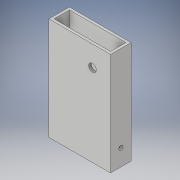
# Autodesk Inventor part: bumper extrusions
Saved by Autodesk Inventor 2019 (Build 230136000, 136)
## iProperties
Created: 2018-12-24
Part Number: bumper extrusions
Material: Generic
Document SubType Name: Modeling
Designer: Tiberus
Density: 1 g/cm^3
Appearance: Default
Author: Tiberus
Autodesk Inventor part; units mm, degrees
ref_plane "YZ Plane" through (0, 0, 0) normal (1, 0, 0) x (0, 1, 0)
ref_plane "XZ Plane" through (0, 0, 0) normal (0, 1, 0) x (-1, 0, 0)
ref_plane "XY Plane" through (0, 0, 0) normal (0, 0, 1) x (1, 0, 0)
sketch "Sketch1" plane through (0, 0, 0) normal (0, 0, 1) x (1, 0, 0)
  line L0 (0, 0) -> (76.2, 0)
  line L1 (76.2, 0) -> (76.2, 127)
  line L2 (76.2, 127) -> (0, 127)
  line L3 (0, 127) -> (0, 0)
  dimension "d0" = 76.2
  dimension "d1" = 127
  constraints: 8 end point, 2 parallel, 1 horizontal, 1 perpendicular
  measures "d0" distance of L2.end L1.end
  measures "d1" distance of L1.end L0.end
extrude "Extrusion1" add sketch "Sketch1" along normal blind 25.4
sketch "Sketch2" plane through (76.2, 0, 0) normal (1, 0, 0) x (0, 0, -1)
  line L0 (0, 0) -> (-25.4, 0) construction
  line L1 (-12.7, 0) -> (-12.7, 20.6502) construction
  circle A0 centre (-12.7, 20.6502) radius 2.5797
  dimension "d4" = 20.6502
  dimension "d5" = 5.1594
  constraints: 2 end point, 1 centre point, 1 coincident, 1 midpoint, 1 vertical
  measures "d4" distance of L1.start L1.end
  measures "d5" diameter of A0
extrude "Extrusion2" cut sketch "Sketch2" against normal blind 762
sketch "Sketch4" plane through (0, 0, 0) normal (0, -1, 0) x (1, 0, 0)
  line L0 (0, 25.4) -> (76.2, 25.4) projected
  line L1 (0, 0) -> (0, 25.4) projected
  line L2 (0, 0) -> (76.2, 0) projected
  line L3 (76.2, 0) -> (76.2, 25.4) projected
  line L4 (73.025, 22.225) -> (3.175, 22.225)
  line L5 (3.175, 22.225) -> (3.175, 3.175)
  line L6 (3.175, 3.175) -> (73.025, 3.175)
  line L7 (73.025, 3.175) -> (73.025, 22.225)
  dimension "d15" = 3.175
  constraints: 8 end point, 3 other
  measures "d15" distance between parallel lines of L0 L4
extrude "Extrusion3" cut sketch "Sketch4" against normal blind 508 contours L7 L6 L5 L4
sketch "Sketch5" plane through (0, 0, 0) normal (-1, 0, 0) x (0, 0, 1)
  line L0 (0, 127) -> (25.4, 127) construction
  line L1 (12.7, 127) -> (12.7, 114.3) construction
  circle A0 centre (12.7, 114.3) radius 2.5797
  point P0 (0, 0)
  dimension "d18" = 12.7
  dimension "d19" = 5.1594
  constraints: 2 end point, 1 centre point, 1 coincident, 1 midpoint, 1 vertical
  measures "d18" distance of L1.start L1.end
  measures "d19" diameter of A0
extrude "Extrusion4" cut sketch "Sketch5" against normal blind 50.8
sketch "Sketch6" plane through (0, 0, 25.4) normal (0, 0, 1) x (1, 0, 0)
  point P0 (53.975, 101.6)
hole "Hole2" at (53.975, 101.6, 25.4) direction (0, 0, -1) diameter 9.525 depth 3.175
sketch "Sketch7" plane through (3.175, 0, 3.175) normal (0, 0, 1) x (1, 0, 0)
  point P0 (50.8, 101.6)
hole "Hole4" at (53.975, 101.6, 3.175) direction (0, 0, -1) diameter 9.525 depth 3.175
body "Solid1"
